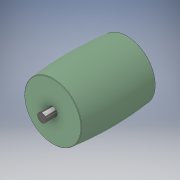
# Autodesk Inventor part: Mechnum small wheel
Saved by Autodesk Inventor 2018 (Build 220112000, 112)
## iProperties
Created: 2018-03-28
Part Number: Mechnum small wheel
Material: Generic
Document SubType Name: Modeling
Designer: Ajith Thomas
Density: 1 g/cm^3
Appearance: Default
Author: Ajith Thomas
Autodesk Inventor part; units mm, degrees
ref_plane "YZ Plane" through (0, 0, 0) normal (1, 0, 0) x (0, 1, 0)
ref_plane "XZ Plane" through (0, 0, 0) normal (0, 1, 0) x (-1, 0, 0)
sketch "Sketch1" plane through (0, 0, 0) normal (1, 0, 0) x (0, 1, 0)
  line L0 (0, 0) -> (0, -8.5)
  line L1 (0, 0) -> (0, 8.5)
  dimension "d0" = 8.5
  dimension "d1" = 8.5
  constraints: 4 end point, 2 vertical
  measures "d0" distance of L0.start L0.end
  measures "d1" distance of L0.start L1.end
ref_plane "Work Plane3" through (0, 0, 0) normal (0, 0, 1) x (1, 0, 0)
ref_plane "Work Plane1" through (0, 0, 8.5) normal (0, 0, 1) x (1, 0, 0)
ref_plane "Work Plane2" through (0, 0, -8.5) normal (0, 0, -1) x (-1, 0, 0)
sketch "Sketch2" plane through (0, 0, 8.5) normal (0, 0, 1) x (1, 0, 0)
  circle A0 centre (0, 0) radius 6.5
  dimension "d2" = 13
  constraints: 1 centre point, 1 coincident
  measures "d2" diameter of A0
sketch "Sketch3" plane through (0, 0, 0) normal (0, 0, 1) x (1, 0, 0)
  circle A0 centre (0, 0) radius 7
  dimension "d3" = 14
  constraints: 1 centre point, 1 coincident
  measures "d3" diameter of A0
sketch "Sketch4" plane through (0, 0, -8.5) normal (0, 0, -1) x (-1, 0, 0)
  circle A0 centre (0, 0) radius 6.5
  dimension "d4" = 13
  constraints: 1 centre point, 1 coincident
  measures "d4" diameter of A0
loft "Loft1" add profiles "Sketch2", "Sketch3", "Sketch4"
fillet "Fillet1" radius 0.1 4 edges at (0, 6.5, 8.5) (0, -6.5, 8.5) (0, 6.5, -8.5) (0, -6.5, -8.5)
sketch "Sketch5" plane through (0.0059, 0.0026, 8.5) normal (0, 0, 1) x (1, 0, 0)
  circle A0 centre (-0.0059, -0.0026) radius 1
  dimension "d12" = 2
  constraints: 1 centre point, 1 coincident
  measures "d12" diameter of A0
extrude "Extrusion1" add sketch "Sketch5" along normal blind 4.2
mirror "Mirror1" about plane through (0, 0, 0) normal (0, 0, 1) of "Extrusion1"
sketch "Sketch6" plane through (0, 0, 12.7) normal (0, 0, 1) x (1, 0, 0)
  circle A0 centre (0, 0) radius 1 projected
extrude "Extrusion2" cut sketch "Sketch6" against normal blind 1.7
sketch "Sketch7" plane through (0, 0, -12.7) normal (0, 0, -1) x (-1, 0, 0)
  circle A0 centre (0, 0) radius 1 projected
extrude "Extrusion3" cut sketch "Sketch7" against normal blind 1.7
body "Solid1"
